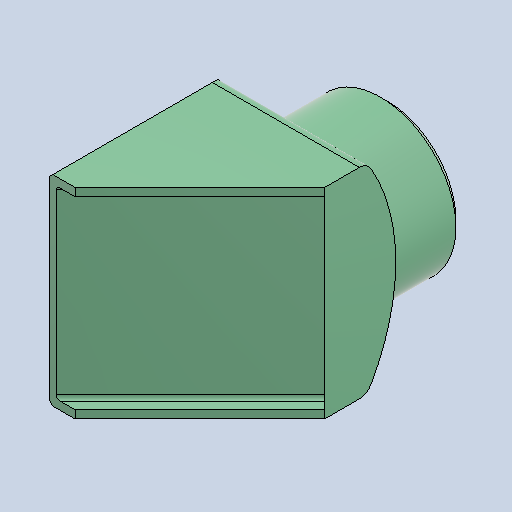
# Autodesk Inventor part: pld-target-holder
Saved by Autodesk Inventor 2026 (Build 300175050, 175E)
## iProperties
Created: 2025-11-13
Part Number: pld-target-holder
Material: ABS Plastic
Document SubType Name: Modeling
Designer: kuzmin
Density: 1.06 g/cm^3
Appearance: Smooth - Dark Sea Green
Author: kuzmin
Autodesk Inventor part; units mm, degrees
ref_plane "YZ Plane" through (0, 0, 0) normal (1, 0, 0) x (0, 1, 0)
ref_plane "XZ Plane" through (0, 0, 0) normal (0, 1, 0) x (-1, 0, 0)
ref_plane "XY Plane" through (0, 0, 0) normal (0, 0, 1) x (1, 0, 0)
sketch "Sketch1" plane through (0, 0, 0) normal (1, 0, 0) x (0, 1, 0)
  circle A0 centre (0, 38.3) radius 28.3
  line L0 (-15, 14.3023) -> (15, 14.3023)
  line L1 (15, 14.3023) -> (15, 39.3023)
  line L2 (15, 39.3023) -> (-15, 39.3023)
  line L3 (-15, 39.3023) -> (-15, 14.3023)
  point P0 (0, 0)
  point P1 (0, 10)
  dimension "d0" = 56.6
  dimension "d1" = 10
  dimension "d2" = 25
  dimension "d3" = 30
  constraints: 8 end point, 3 point on circle, 2 parallel, 2 vertical alignment, 1 centre point, 1 horizontal, 1 perpendicular
  measures "d0" diameter of A0
  measures "d1" distance of point (0, 0) A0.start
  measures "d2" distance of L0.end L1.end
  measures "d3" distance of L1.end L2.end
extrude "Extrusion1" add sketch "Sketch1" along normal mid plane 22.5 contours L0 A0 | L3 L2 L1 L0
sketch "Sketch2" plane through (0, 0, 0) normal (0, 0, 1) x (1, 0, 0)
  circle A0 centre (0, 0) radius 11.25
  dimension "d6" = 22.5
  constraints: 1 centre point, 1 coincident
  measures "d6" diameter of A0
extrude "Extrusion2" add sketch "Sketch2" along normal up to surface
sketch "Sketch3" plane through (-11.25, 0, 14.3023) normal (0, -1, 0) x (1, 0, 0)
  line L0 (0, 25) -> (22.5, 25) projected
  line L1 (22.5, 25) -> (22.5, 0) projected
  line L2 (1, 25) -> (22.5, 3.5)
  line L3 (22.5, 6.3284) -> (21.0858, 4.9142)
  line L4 (0, 0) -> (0, 25) projected
  point P0 (11.25, -14.3023)
  dimension "d12" = 45
  dimension "d13" = 1
  dimension "d14" = 2
  constraints: 4 end point, 4 point on line, 1 perpendicular
  measures "d12" angle of L0 L2
  measures "d13" distance from line of L4 L2.start
  measures "d14" distance of L3.start L3.end
extrude "Extrusion3" cut sketch "Sketch3" along normal mid plane 27.6 contours L0 L1 L3 L2
sketch "Sketch4" plane through (0, 0, 0) normal (0, 1, 0) x (-1, 0, 0)
  line L0 (-11.25, 14.3023) -> (-11.25, 39.3023) projected
  line L1 (-11.25, 20.6307) -> (7.4216, 39.3023)
  line L2 (10.25, 39.3023) -> (-11.25, 39.3023) projected
  line L3 (-9.8358, 19.2165) -> (10.25, 39.3023) projected
  point P0 (0, 0)
  constraints: 2 end point, 1 parallel, 1 point on line
extrude "Extrusion4" cut sketch "Sketch4" along normal through all both and the other way through all
fillet "Fillet1" radius 0.5 2 edges at (-0.2071, 13.8, 29.2594) (-0.2071, -13.8, 29.2594)
chamfer "Chamfer1" distance 1 angle 45 1 edges at (-11.25, 0, 0)
chamfer "Chamfer2" distance 0.5 angle 45 2 edges at (-11.25, 15, 26.8023) (-11.25, -15, 26.8023)
fillet "Fillet2" radius 2 2 edges at (0.25, -15, 14.3023) (0.25, 15, 14.3023)
equation "\"d3\" = width"
equation "\"d10\" = sample_cut"
equation "\"width\" = 30"
equation "\"sample_cut\" = 27.6"
body "Solid1"
